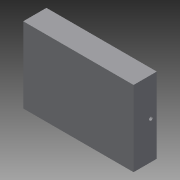
# Autodesk Inventor part: RESONATORCHAMBER
Saved by Autodesk Inventor 2013 (Build 170138000, 138)
## iProperties
Created: 2013-06-23
Part Number: RESONATORCHAMBER
Material: Generic
Document SubType Name: Modeling
Designer: Virtual
Density: 1 g/cm^3
Author: Virtual
Autodesk Inventor part; units mm, degrees
ref_plane "YZ Plane" through (0, 0, 0) normal (1, 0, 0) x (0, 1, 0)
ref_plane "XZ Plane" through (0, 0, 0) normal (0, 1, 0) x (-1, 0, 0)
ref_plane "XY Plane" through (0, 0, 0) normal (0, 0, 1) x (1, 0, 0)
sketch "Sketch1" plane through (0, 0, 0) normal (0, 1, 0) x (-1, 0, 0)
  line L0 (0, 0) -> (95, 0)
  line L1 (95, 0) -> (95, 65)
  line L2 (95, 65) -> (0, 65)
  line L3 (0, 65) -> (0, 0)
  constraints: 8 end point, 2 parallel, 1 horizontal, 1 perpendicular
extrude "Extrusion1" add sketch "Sketch1" along normal blind 20
sketch "Sketch2" plane through (0, 20, 0) normal (0, 1, 0) x (1, 0, 0)
  line L0 (-5, -5) -> (-90, -5)
  line L1 (-90, -5) -> (-90, -60)
  line L2 (-90, -60) -> (-5, -60)
  line L3 (-5, -60) -> (-5, -5)
  constraints: 8 end point, 2 parallel, 1 horizontal, 1 perpendicular
extrude "Extrusion2" cut sketch "Sketch2" against normal blind 15
sketch "Sketch3" plane through (-95, 0, 0) normal (-1, 0, 0) x (0, 0, 1)
  circle A0 centre (32.5, 15) radius 1.625
  dimension "d4" = 3.25
  constraints: 1 centre point
  measures "d4" diameter of A0
hole "Hole1" at (-95, 15, 32.5) direction (1, 0, 0) diameter 3.25 end through all
body "Solid1"
